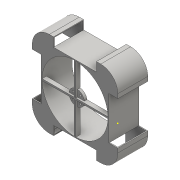
# Autodesk Inventor part: Motor mount (plain)
Saved by Autodesk Inventor 2016 (Build 200138000, 138)
## iProperties
Created: 2016-03-10
Part Number: Motor mount (plain)
Material: Generic
Document SubType Name: Modeling
Designer: s_sud
Density: 1 g/cm^3
Appearance: Default
Author: s_sud
Autodesk Inventor part; units mm, degrees
ref_plane "YZ Plane" through (0, 0, 0) normal (1, 0, 0) x (0, 1, 0)
ref_plane "XZ Plane" through (0, 0, 0) normal (0, 1, 0) x (-1, 0, 0)
ref_plane "XY Plane" through (0, 0, 0) normal (0, 0, 1) x (1, 0, 0)
sketch "Sketch1" plane through (0, 0, 0) normal (0, 1, 0) x (-1, 0, 0)
  circle A0 centre (0, 0) radius 38.5
  circle A1 centre (0, 0) radius 39
  dimension "d0" = 77
  dimension "d1" = 78
  constraints: 2 centre point, 2 coincident
  measures "d0" diameter of A0
  measures "d1" diameter of A1
extrude "Extrusion1" add sketch "Sketch1" along normal blind 35
sketch "Sketch24" plane through (0, 35, 0) normal (0, 1, 0) x (1, 0, 0)
  line L0 (-39.5, -39.5) -> (39.5, -39.5)
  line L1 (39.5, -39.5) -> (39.5, 39.5)
  line L2 (39.5, 39.5) -> (-39.5, 39.5)
  line L3 (-39.5, 39.5) -> (-39.5, -39.5)
  line L4 (50, -50) -> (-50, -50)
  line L5 (-50, -50) -> (-50, 50)
  line L6 (-50, 50) -> (50, 50)
  line L7 (50, 50) -> (50, -50)
  line L8 (50, -50) -> (-50, 50) construction
  line L9 (-50, -50) -> (50, 50) construction
  line L10 (-25, -50) -> (-25, -39.5)
  line L11 (25, -50) -> (25, -39.5)
  line L12 (-50, -25) -> (-39.5, -25)
  line L13 (-50, 25) -> (-39.5, 25)
  line L14 (-25, 39.5) -> (-25, 50)
  line L15 (25, 39.5) -> (25, 50)
  line L16 (39.5, -25) -> (50, -25)
  line L17 (39.5, 25) -> (50, 25)
  line L18 (38.5, -38.5) -> (-38.5, -38.5)
  line L19 (-38.5, -38.5) -> (-38.5, 38.5)
  line L20 (-38.5, 38.5) -> (38.5, 38.5)
  line L21 (38.5, 38.5) -> (38.5, -38.5)
  line L22 (38.5, -38.5) -> (-38.5, 38.5) construction
  line L23 (-38.5, -38.5) -> (38.5, 38.5) construction
  line L24 (0, -50) -> (0, -39.5)
  line L25 (-50, 0) -> (-39.5, 0)
  line L26 (0, -38.5) -> (0, 38.5)
  line L27 (0, 39.5) -> (0, 50)
  line L28 (-38.5, 0) -> (38.5, 0)
  line L29 (39.5, 0) -> (50, 0)
  point P0 (0, 0)
  point P1 (50, 50)
  point P2 (50, -50)
  dimension "d137" = 0
  dimension "d165" = 77
  dimension "d166" = 77
  dimension "d167" = 38.5
  dimension "d168" = 38.5
  dimension "d169" = 38.5
  dimension "d170" = 79
  dimension "d171" = 79
  dimension "d172" = 39.5
  dimension "d173" = 39.5
  dimension "d174" = 39.5
  dimension "d175" = 100
  dimension "d176" = 25
  dimension "d177" = 25
  dimension "d178" = 25
  dimension "d179" = 25
  dimension "d180" = 25
  dimension "d181" = 25
  dimension "d182" = 25
  dimension "d183" = 25
  dimension "d184" = 50
  constraints: 60 end point, 25 point on line, 16 midpoint, 11 perpendicular, 7 horizontal, 6 parallel, 4 vertical, 16 other
  measures "d165" distance of L18.start L18.end
  measures "d166" distance of L18.end L19.end
  measures "d167" distance between parallel lines of L28 L18
  measures "d168" distance between parallel lines of L20 L28
  measures "d169" distance between parallel lines of L26 L19
  measures "d170" distance of L2.end L0.start
  measures "d171" distance of L0.start L0.end
  measures "d172" distance between parallel lines of L3 L26
  measures "d173" distance between parallel lines of L1 L26
  measures "d174" distance between parallel lines of L28 L2
  measures "d175" distance of L5.start L5.end
  measures "d176" distance between parallel lines of L10 L24
  measures "d177" distance between parallel lines of L24 L11
  measures "d178" distance between parallel lines of L25 L12
  measures "d179" distance between parallel lines of L13 L25
  measures "d180" distance between parallel lines of L27 L14
  measures "d181" distance between parallel lines of L27 L15
  measures "d182" distance between parallel lines of L17 L29
  measures "d183" distance between parallel lines of L29 L16
  measures "d184" distance between parallel lines of L5 L24
extrude "Extrusion24" add sketch "Sketch24" against normal blind 35 contours L3 L2 L1 L0 | L0 L10 L4 L5 L12 L3 | L0 L1 L16 L7 L4 L11 | L13 L5 L6 L14 L2 L3 | L1 L2 L15 L6 L7 L17
fillet "Fillet4" radius 20 4 edges at (50, 17.5, -50) (-50, 17.5, -50) (-50, 17.5, 50) (50, 17.5, 50)
sketch "Sketch27" plane through (0, 35, 0) normal (0, 1, 0) x (1, 0, 0)
  circle A0 centre (0, 0) radius 38.5
  line L0 (-6.2249, 38.5) -> (-38.5, 38.5) projected
  line L1 (38.5, -38.5) -> (-38.5, -38.5)
  line L2 (-38.5, -38.5) -> (-38.5, 38.5)
  line L3 (-38.5, 38.5) -> (38.5, 38.5)
  line L4 (38.5, 38.5) -> (38.5, -38.5)
  line L5 (38.5, -38.5) -> (-38.5, 38.5) construction
  line L6 (-38.5, -38.5) -> (38.5, 38.5) construction
  dimension "d186" = 77
  constraints: 12 end point, 2 midpoint, 2 parallel, 1 centre point, 1 coincident, 1 horizontal, 1 perpendicular
  measures "d186" diameter of A0
extrude "Extrusion26" add sketch "Sketch27" against normal blind 35 contours L4 L1 A0 | A0 L3 L4 | A0 L2 L0 L3 | L1 L2 A0
shell "Shell4" thickness 1 removed faces 8 at (25, 23.3333, -46.5) at (43, 23.3333, -25) at (46.5, 23.3333, 25) at (25, 11.6667, 43) at (-25, 11.6667, 46.5) at (-43, 11.6667, 25) at (-25, 11.6667, -43) at (-46.5, 23.3333, -25)
sketch "Sketch30" plane through (50, 35, 30) normal (1, 0, 0) x (0, 0, -1)
  point P0 (30, -35)
sketch "Sketch33" plane through (0, 0, 0) normal (0, -1, 0) x (1, 0, 0)
  line L0 (1, 39) -> (-1, 39)
  line L1 (-1, 39) -> (-1, -39)
  line L2 (-1, -39) -> (1, -39)
  line L3 (1, -39) -> (1, 39)
  line L4 (1, 39) -> (-1, -39) construction
  line L5 (-1, 39) -> (1, -39) construction
  line L6 (39, 1) -> (-39, 1)
  line L7 (-39, 1) -> (-39, -1)
  line L8 (-39, -1) -> (39, -1)
  line L9 (39, -1) -> (39, 1)
  line L10 (39, 1) -> (-39, -1) construction
  line L11 (-39, 1) -> (39, -1) construction
  point P0 (0, 0)
  dimension "d199" = 78
  dimension "d200" = 2
  dimension "d201" = 78
  dimension "d202" = 2
  constraints: 24 end point, 4 midpoint, 4 parallel, 2 horizontal, 2 perpendicular
  measures "d199" distance of L0.end L1.end
  measures "d200" distance of L1.end L2.end
  measures "d201" distance of L7.end L8.end
  measures "d202" distance of L8.end L6.start
extrude "Extrusion29" add sketch "Sketch33" against normal blind 5
sketch "Sketch34" plane through (0, 5, 0) normal (0, 1, 0) x (1, 0, 0)
  circle A0 centre (0, 0) radius 9
  circle A1 centre (0, 6) radius 1
  circle A2 centre (-4.2426, 4.2426) radius 1
  circle A3 centre (-6, 0) radius 1
  circle A4 centre (-4.2426, -4.2426) radius 1
  circle A5 centre (0, -6) radius 1
  circle A6 centre (4.2426, -4.2426) radius 1
  circle A7 centre (6, 0) radius 1
  circle A8 centre (4.2426, 4.2426) radius 1
  dimension "d205" = 18
  dimension "d206" = 2
  dimension "d207" = 6
  dimension "d210" = 360
  constraints: 9 centre point, 1 coincident, 17 other
  measures "d205" diameter of A0
  measures "d206" diameter of A1
  measures "d207" distance of A1.centre point (0, 0)
extrude "Extrusion30" add sketch "Sketch34" against normal blind 3
body "Solid1"
